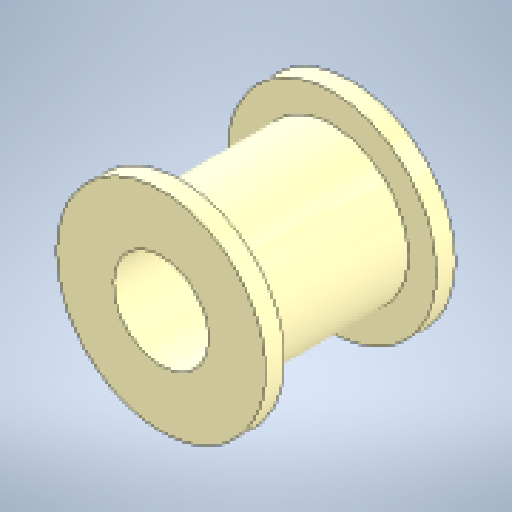
# Autodesk Inventor part: Spring Anchor
Saved by Autodesk Inventor 2023.2 (Build 272271000, 271)
## iProperties
Created: 2024-03-17
Part Number: Spring Anchor
Material: Nylon 6/6
Document SubType Name: Modeling
Designer: Nathan Cai
Density: 1.13 g/cm^3
Appearance: Nylon 6
Author: Nathan Cai
Autodesk Inventor part; units mm, degrees
ref_plane "YZ Plane" through (0, 0, 0) normal (1, 0, 0) x (0, 1, 0)
ref_plane "XZ Plane" through (0, 0, 0) normal (0, 1, 0) x (-1, 0, 0)
ref_plane "XY Plane" through (0, 0, 0) normal (0, 0, 1) x (1, 0, 0)
sketch "Sketch1" plane through (0, 0, 0) normal (1, 0, 0) x (0, 1, 0)
  line L0 (0, 0) -> (3.9688, 0) construction
  line L1 (3.9688, 0) -> (3.9687, 19.05)
  line L2 (3.9687, 19.05) -> (0, 19.05) construction
  line L3 (0, 19.05) -> (0, 0) construction
  line L4 (3.9688, 0) -> (6.35, 0)
  line L5 (6.35, 0) -> (6.35, 19.05)
  line L6 (6.35, 19.05) -> (3.9687, 19.05)
  line L7 (3.9687, 19.05) -> (3.9688, 0)
  line L8 (6.35, 0) -> (8.7313, 0)
  line L9 (8.7313, 0) -> (8.7312, 6.35)
  line L10 (8.7312, 6.35) -> (6.35, 6.35)
  line L11 (6.35, 6.35) -> (6.35, 0)
  line L12 (6.35, 19.05) -> (8.7312, 19.05)
  line L13 (8.7312, 19.05) -> (8.7312, 15.875)
  line L14 (8.7312, 15.875) -> (6.35, 15.875)
  line L15 (6.35, 15.875) -> (6.35, 19.05)
  point P0 (6.35, 6.35)
  point P1 (6.35, 15.875)
  dimension "d0" = 3.9688
  dimension "d1" = 19.05
  dimension "d2" = 2.3813
  dimension "d3" = 2.3813
  dimension "d4" = 6.35
  dimension "d5" = 2.3813
  dimension "d8" = 9.525
  constraints: 32 end point, 8 parallel, 4 horizontal, 4 perpendicular, 1 point on line
  measures "d0" distance of L2.end L1.end
  measures "d1" distance between parallel lines of L0 L2
  measures "d2" distance of L6.end L5.end
  measures "d3" distance of L10.end L9.end
  measures "d4" distance of L9.end L8.end
  measures "d5" distance of L13.end L14.end
  measures "d8" distance between parallel lines of L10 L14
revolve "Revolution1" add sketch "Sketch1" angle 360 about axis through (0, 0, 19.05) along (0, 0, -1)
chamfer "Chamfer1" distance 0.5 angle 45 3 edges at (0, -8.7313, 0) (0, -8.7312, 6.35) (0, -8.7312, 15.875)
equation "\"d5\" = d3"
body "Solid1"
